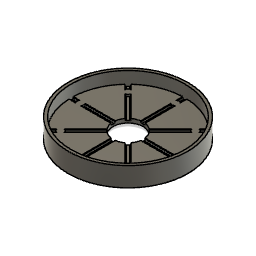
Fusion File (Autodesk Fusion 360 design; units mm, degrees)
Autodesk Fusion 360 part; units mm, degrees
sketch "Sketch2" plane through (0, 0, 0) normal (1, 0, 0) x (0, 0, -1)
  line L0 (0, 0) -> (0, 16)
  line L1 (-49.5, 3.3) -> (-12.45, 3.3)
  line L2 (-12.45, 3.3) -> (-12.45, 0)
  line L3 (-12.45, 0) -> (-49.5, 0)
  line L4 (-49.5, 0) -> (-49.5, 3.3)
  line L5 (-49.5, 0) -> (-45.3, 0)
  line L6 (-45.3, 0) -> (-45.3, -2.8)
  line L7 (-45.3, -2.8) -> (-49.5, -2.8)
  line L8 (-49.5, -2.8) -> (-49.5, 0)
  line L9 (-23.5, 0) -> (-20.4, 0)
  line L10 (-20.4, 0) -> (-20.4, -2.8)
  line L11 (-20.4, -2.8) -> (-23.5, -2.8)
  line L12 (-23.5, -2.8) -> (-23.5, 0)
  line L13 (-49.5, 13.2) -> (-47.1, 13.2)
  line L14 (-47.1, 13.2) -> (-47.1, 3.3)
  line L15 (-47.1, 3.3) -> (-49.5, 3.3)
  line L16 (-49.5, 3.3) -> (-49.5, 13.2)
  dimension "d2" = 16
  dimension "d3" = 37.05
  dimension "d4" = 3.3
  dimension "d5" = 12.45
  dimension "d6" = 3.3
  dimension "d7" = 4.2
  dimension "d8" = 2.8
  dimension "d9" = 3.1
  dimension "d10" = 2.8
  dimension "d11" = 7.95
  dimension "d12" = 2.4
  dimension "d13" = 9.9
  constraint coincident L0.start origin
  constraint vertical L0
  constraint horizontal L1
  constraint vertical L2
  constraint horizontal L3
  constraint vertical L4
  constraint horizontal L5
  constraint vertical L6
  constraint horizontal L7
  constraint vertical L8
  constraint coincident L3.end L4.start
  constraint horizontal L9
  constraint vertical L10
  constraint horizontal L11
  constraint vertical L12
  constraint coincident L3 L9.end
  constraint horizontal L13
  constraint vertical L14
  constraint horizontal L15
  constraint vertical L16
  constraint coincident L1.start L4.end
  measures "d2" distance of L0.start L0.end
  measures "d3" distance of L1.start L1.end
  measures "d4" distance of L1.start L3.end
  measures "d5" horizontal distance of L0.start L2.end
  measures "d6" vertical distance of L0.start L1.end
  measures "d7" distance of L3.end L5.end
  measures "d8" distance of L5.end L6.end
  measures "d9" distance of L9.start L9.end
  measures "d10" distance of L9.start L11.end
  measures "d11" horizontal distance of L2.end L9.end
  measures "d12" distance of L13.start L13.end
  measures "d13" distance of L13.start L1.start
revolve "Revolve1" add sketch "Sketch2" angle 360 about axis through (0, 0, 0) along (0, 1, 0) makes body 1
sketch "Sketch3" plane through (0, 0, 0) normal (0, -1, 0) x (1, 0, 0)
  circle A0 centre (0, 0) radius 23.5
  circle A1 centre (0, 0) radius 45.3
  line L0 (23.5, -23.5) -> (-23.5, -23.5)
  line L1 (-23.5, -23.5) -> (-23.5, 23.5)
  line L2 (-23.5, 23.5) -> (23.5, 23.5)
  line L3 (23.5, 23.5) -> (23.5, -23.5)
  line L4 (-23.5, -23.5) -> (23.5, 23.5)
  line L5 (1.4, 23.5) -> (-1.4, 23.5)
  line L6 (-1.4, 23.5) -> (-1.4, 45.3)
  line L7 (-1.4, 45.3) -> (1.4, 45.3)
  line L8 (1.4, 45.3) -> (1.4, 23.5)
  line L9 (-1.4, 25) -> (1.4, 25)
  line L10 (1.4, 25) -> (1.4, 22)
  line L11 (1.4, 22) -> (-1.4, 22)
  line L12 (-1.4, 22) -> (-1.4, 25)
  line L13 (1.4, 25) -> (-1.4, 22)
  point P0 (0, 23.5)
  dimension "d17" = 47
  dimension "d18" = 47
  dimension "d19" = 2.8
  dimension "d20" = 21.8
  dimension "d36" = 2.8
  dimension "d37" = 3
  constraint horizontal L0
  constraint vertical L1
  constraint horizontal L2
  constraint vertical L3
  constraint midpoint A0.centre L4
  constraint horizontal L5
  constraint vertical L6
  constraint horizontal L7
  constraint vertical L8
  constraint midpoint L5 P0
  constraint midpoint L2 P0
  constraint horizontal L9
  constraint vertical L10
  constraint horizontal L11
  constraint vertical L12
  constraint coincident L6 L9.start
  constraint midpoint P0 L13
  measures "d17" distance of L0.start L0.end
  measures "d18" distance of L0.start L2.end
  measures "d19" distance of L5.start L5.end
  measures "d20" distance of L5.start L7.end
  measures "d36" distance of L9.start L9.end
  measures "d37" distance of L9.start L11.end
extrude "Extrude1" add sketch "Sketch3" along normal blind 2.8 separate body contours A0 L2 L5 L10 | L2 L5 L8 L10 L13 | A0 L2 L5 L12 | L2 L5 L6 L9 L12 L13 | A1 L6 L8 L9 makes body 2
pattern_circular "C-Pattern1" count 8 over 360 about axis through (0, -2.8, 0) along (0, 1, 0) of bodies 2 makes body 3 at (22.4624, 0, 22.4624) makes body 4 at (31.7667, 0, 0) makes body 5 at (22.4624, 0, -22.4624) makes body 6 at (0, 0, -31.7667) makes body 7 at (-22.4624, 0, -22.4624) makes body 8 at (-31.7667, 0, 0) makes body 9 at (-22.4624, 0, 22.4624)
sketch "Sketch4" plane through (0, 3.3, 0) normal (0, 1, 0) x (-1, 0, 0)
  circle A0 centre (0, 0) radius 47.1
  circle A1 centre (0, 0) radius 12.45
  line L0 (12.45, -12.45) -> (-12.45, -12.45)
  line L1 (-12.45, -12.45) -> (-12.45, 12.45)
  line L2 (-12.45, 12.45) -> (12.45, 12.45)
  line L3 (12.45, 12.45) -> (12.45, -12.45)
  line L4 (-12.45, -12.45) -> (12.45, 12.45)
  line L5 (1.725, 12.45) -> (-1.725, 12.45)
  line L6 (-1.725, 12.45) -> (-1.725, 47.1)
  line L7 (-1.725, 47.1) -> (1.725, 47.1)
  line L8 (1.725, 47.1) -> (1.725, 12.45)
  circle A2 centre (0, 39.55) radius 2.8
  line L9 (1.725, 10.45) -> (-1.725, 10.45)
  line L10 (-1.725, 10.45) -> (-1.725, 14.45)
  line L11 (-1.725, 14.45) -> (1.725, 14.45)
  line L12 (1.725, 14.45) -> (1.725, 10.45)
  line L13 (-1.725, 10.45) -> (1.725, 14.45)
  point P0 (0, 12.45)
  dimension "d25" = 24.9
  dimension "d26" = 24.9
  dimension "d27" = 3.45
  dimension "d28" = 34.65
  dimension "d29" = 5.6
  dimension "d30" = 27.1
  dimension "d31" = 12.45
  dimension "d34" = 3.45
  dimension "d35" = 4
  constraint horizontal L0
  constraint vertical L1
  constraint horizontal L2
  constraint vertical L3
  constraint midpoint A0.centre L4
  constraint horizontal L5
  constraint vertical L6
  constraint horizontal L7
  constraint vertical L8
  constraint midpoint L5 P0
  constraint midpoint L2 P0
  constraint horizontal L9
  constraint vertical L10
  constraint horizontal L11
  constraint vertical L12
  constraint midpoint P0 L13
  measures "d25" distance of L0.start L0.end
  measures "d26" distance of L0.start L2.end
  measures "d27" distance of L5.start L5.end
  measures "d28" distance of L5.start L7.end
  measures "d29" diameter of A2
  measures "d30" vertical distance of P0 A2.centre
  measures "d31" horizontal distance of L1.end A2.centre
  measures "d34" distance of L9.start L9.end
  measures "d35" distance of L9.start L11.end
extrude "Extrude2" cut sketch "Sketch4" against normal blind 1.55 contours A0 L6 L8 A2 | L6 L8 A2 L11 | L2 L5 L6 L10 L11 L13 | L2 L5 L8 L12 L13 | A1 L2 L5 L12 | A1 L10 L13 | A1 L2 L5 L10 | A1 L9 L12 L13 bodies 1
fillet "Fillet3" radius 0.8 4 edges at (1.725, 1.75, 24.8372) (1.725, 1.75, 44.412) (-1.725, 1.75, 24.8372) (-1.725, 1.75, 44.412) on bodies 1
pattern_circular "C-Pattern3" count 8 over 360 about axis through (0, 13.2, 0) along (0, 1, 0) of 12 faces at (0.9855, 1.7523, 45.4492) (0.0628, 1.75, 45.5139) (-0.9855, 1.7523, 45.4492) (-1.725, 3.05, 45.2974) (-1.725, 3.05, 20.6681) (-1.6602, 2.2346, 20.6597) (0.8512, 2.7833, 36.8825) (0.8512, 2.7833, 42.2175) (1.725, 3.05, 43.5265) (1.2774, 1.8318, 28.8403) (1.725, 3.05, 29.0063) (0, 1.75, 28.6542) on bodies 1
